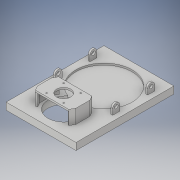
# Autodesk Inventor part: base
Saved by Autodesk Inventor 2019 (Build 230136000, 136)
## iProperties
Created: 2019-05-15
Part Number: base
Material: Generic
Document SubType Name: Modeling
Designer: Nathan
Density: 1 g/cm^3
Appearance: Default
Author: Nathan
Autodesk Inventor part; units mm, degrees
ref_plane "YZ Plane" through (0, 0, 0) normal (1, 0, 0) x (0, 1, 0)
ref_plane "XZ Plane" through (0, 0, 0) normal (0, 1, 0) x (-1, 0, 0)
ref_plane "XY Plane" through (0, 0, 0) normal (0, 0, 1) x (1, 0, 0)
sketch "Sketch1" plane through (0, 0, 0) normal (0, 1, 0) x (-1, 0, 0)
  line L0 (63.5, 88.9) -> (-63.5, 88.9)
  line L1 (-63.5, 88.9) -> (-63.5, -88.9)
  line L2 (-63.5, -88.9) -> (63.5, -88.9)
  line L3 (63.5, -88.9) -> (63.5, 88.9)
  line L4 (63.5, 88.9) -> (-63.5, -88.9) construction
  line L5 (-63.5, 88.9) -> (63.5, -88.9) construction
  point P0 (0, 0)
  dimension "d0" = 127
  dimension "d1" = 177.8
  constraints: 12 end point, 2 midpoint, 2 parallel, 1 horizontal, 1 perpendicular
  measures "d0" distance of L2.end L1.end
  measures "d1" distance of L1.end L0.end
extrude "Extrusion1" add sketch "Sketch1" along normal blind 12.7
sketch "Sketch2" plane through (0, 12.7, 0) normal (0, 1, 0) x (1, 0, 0)
  circle A0 centre (0, 25.4) radius 51.0159
  line L0 (-63.5, 88.9) -> (-63.5, -88.9) projected
  line L1 (63.5, 88.9) -> (-63.5, 88.9) projected
  point P0 (0, 0)
  dimension "d4" = 102.0318
  dimension "d5" = 63.5
  dimension "d6" = 63.5
  constraints: 1 centre point
  measures "d4" diameter of A0
  measures "d5" distance from line of L0 A0.centre
  measures "d6" distance from line of L1 A0.centre
sketch "Sketch3" plane through (0, 12.7, 0) normal (0, 1, 0) x (1, 0, 0)
  arc A0 (-24.2412, -32.7116) -> (24.2412, -32.7116) centre (0, -47.8409) ccw
  line L0 (-24.2412, -32.7116) -> (-17.8095, -22.4063)
  line L1 (0, 124.46) -> (0, -124.46) projected
  line L2 (24.2412, -32.7116) -> (17.8095, -22.4063)
  arc A1 (17.8095, -22.4063) -> (-17.8095, -22.4063) centre (0, -33.5215) ccw
  circle A2 centre (0, -47.8409) radius 22.225 construction
  circle A3 centre (0, 25.4) radius 51.0159 projected
  point P0 (0, 0)
  dimension "d13" = 57.15
  dimension "d14" = 70
  dimension "d58" = 44.45
  constraints: 4 end point, 4 point on circle, 3 centre point, 2 symmetric about line, 2 tangent, 1 coincident, 1 point on line, 1 vertical alignment, 1 other
  measures "d13" diameter of A0
  measures "d58" diameter of A2
extrude "Extrusion3" cut sketch "Sketch3" against normal through all contours L0 A3 L1 A0 | L1 A3 L2 A0 | A1 L1 A3 | L1 A1 A3 picked at (-3.4245, -21.2764) picked at (3.4245, -21.2764)
sketch "Sketch5" plane through (0, 12.7, 0) normal (0, 1, 0) x (1, 0, 0)
  line L0 (-34.925, -35.1409) -> (-30.2521, -26.8409)
  line L1 (-30.2521, -26.8409) -> (-27.4855, -28.3985)
  line L2 (-27.4855, -28.3985) -> (-31.75, -35.9732)
  line L3 (-31.75, -35.9732) -> (-31.75, -59.7086)
  line L4 (-31.75, -59.7086) -> (-27.4855, -67.2833)
  line L5 (-27.4855, -67.2833) -> (-30.2521, -68.8409)
  line L6 (-34.925, -35.1409) -> (-34.925, -60.5409)
  line L7 (-34.925, -60.5409) -> (-30.2521, -68.8409)
  arc A0 (-24.2412, -32.7116) -> (24.2412, -32.7116) centre (0, -47.8409) ccw projected
  arc A1 (-24.2412, -32.7116) -> (24.2412, -32.7116) centre (0, -47.8409) ccw construction
  line L8 (-28.575, -47.8409) -> (28.575, -47.8409) construction
  line L9 (0, 124.46) -> (0, -124.46) construction
  line L10 (34.925, -35.1409) -> (30.2521, -26.8409)
  line L11 (30.2521, -26.8409) -> (27.4855, -28.3985)
  line L12 (27.4855, -28.3985) -> (31.75, -35.9732)
  line L13 (31.75, -35.9732) -> (31.75, -59.7086)
  line L14 (31.75, -59.7086) -> (27.4855, -67.2833)
  line L15 (27.4855, -67.2833) -> (30.2521, -68.8409)
  line L16 (34.925, -35.1409) -> (34.925, -60.5409)
  line L17 (34.925, -60.5409) -> (30.2521, -68.8409)
  point P0 (0, 0)
  point P1 (-31.75, -47.8409)
  point P2 (31.75, -47.8409)
  dimension "d16" = 3.175
  dimension "d17" = 3.175
  dimension "d18" = 3.175
  dimension "d19" = 42
  dimension "d20" = 25.4
  dimension "d21" = 9.525
  dimension "d22" = 63.5
  constraints: 34 end point, 9 symmetric about line, 3 parallel, 2 midpoint, 2 point on circle, 1 coincident, 1 horizontal, 1 horizontal alignment, 1 perpendicular, 1 vertical, 2 other
  measures "d16" distance between parallel lines of L6 L3
  measures "d17" distance between parallel lines of L2 L0
  measures "d18" distance between parallel lines of L7 L4
  measures "d19" distance of L5.end L0.end
  measures "d20" distance of L0.start L6.end
  measures "d21" distance of L0.start L0.end
  measures "d22" distance between parallel lines of L13 L3
extrude "Extrusion4" add sketch "Sketch5" along normal blind 25.4
sketch "Sketch6" plane through (0, 38.1, 0) normal (0, 1, 0) x (1, 0, 0)
  line L0 (-30.2521, -68.8409) -> (-27.4855, -67.2833) projected
  line L1 (27.4855, -67.2833) -> (30.2521, -68.8409) projected
  line L2 (31.75, -59.7086) -> (27.4855, -67.2833) projected
  line L3 (31.75, -35.9732) -> (31.75, -59.7086) projected
  line L4 (27.4855, -28.3985) -> (31.75, -35.9732) projected
  line L5 (30.2521, -26.8409) -> (27.4855, -28.3985) projected
  line L6 (-27.4855, -28.3985) -> (-30.2521, -26.8409) projected
  line L7 (-31.75, -35.9732) -> (-27.4855, -28.3985) projected
  line L8 (-31.75, -59.7086) -> (-31.75, -35.9732) projected
  line L9 (-27.4855, -67.2833) -> (-31.75, -59.7086) projected
  line L10 (-30.2521, -68.8409) -> (30.2521, -68.8409)
  line L11 (30.2521, -26.8409) -> (-30.2521, -26.8409)
  point P0 (0, 0)
  constraints: 4 end point, 1 horizontal, 1 parallel
extrude "Extrusion5" add sketch "Sketch6" against normal blind 3.175
sketch "Sketch7" plane through (0, 38.1, 0) normal (0, 1, 0) x (1, 0, 0)
  arc A0 (-24.2412, -32.7116) -> (24.2412, -32.7116) centre (0, -47.8409) ccw projected
  line L0 (21, -68.8409) -> (-21, -68.8409) construction
  line L1 (-21, -68.8409) -> (-21, -26.8409) construction
  line L2 (-21, -26.8409) -> (21, -26.8409) construction
  line L3 (21, -26.8409) -> (21, -68.8409) construction
  line L4 (21, -68.8409) -> (-21, -26.8409) construction
  line L5 (-21, -68.8409) -> (21, -26.8409) construction
  line L6 (15.5, -63.3409) -> (-15.5, -63.3409) construction
  line L7 (-15.5, -63.3409) -> (-15.5, -32.3409) construction
  line L8 (-15.5, -32.3409) -> (15.5, -32.3409) construction
  line L9 (15.5, -32.3409) -> (15.5, -63.3409) construction
  line L10 (15.5, -63.3409) -> (-15.5, -32.3409) construction
  line L11 (-15.5, -63.3409) -> (15.5, -32.3409) construction
  circle A1 centre (0, -47.8409) radius 12.7
  point P0 (0, 0)
  dimension "d27" = 42
  dimension "d28" = 42
  dimension "d29" = 31
  dimension "d30" = 31
  dimension "d31" = 25.4
  constraints: 24 end point, 5 coincident, 4 midpoint, 4 parallel, 2 horizontal, 2 perpendicular, 1 centre point
  measures "d27" distance of L1.end L2.end
  measures "d28" distance of L0.end L1.end
  measures "d29" distance of L7.end L8.end
  measures "d30" distance of L6.end L7.end
  measures "d31" diameter of A1
extrude "Extrusion6" cut sketch "Sketch7" against normal through all
hole "Hole1" at (-15.5, 38.1, 63.3409) at (15.5, 38.1, 63.3409) at (15.5, 38.1, 32.3409) at (-15.5, 38.1, 32.3409) direction (0, -1, 0) diameter 2.5 depth 3.175 tip angle 118
sketch "Sketch8" plane through (0, 12.7, 0) normal (0, 1, 0) x (1, 0, 0)
  line L0 (-53.975, -12.7) -> (-50.8, -12.7)
  line L1 (-50.8, -12.7) -> (-50.8, 0)
  line L2 (-50.8, 0) -> (-53.975, 0)
  line L3 (-53.975, 0) -> (-53.975, -12.7)
  line L4 (-51.0159, 25.4) -> (51.0159, 25.4) construction
  line L5 (0, -25.6159) -> (0, 76.4159) construction
  point P0 (0, 0)
  point P1 (0, 25.4)
  point P2 (0, 25.4)
  dimension "d41" = 12.7
  dimension "d42" = 3.175
  dimension "d43" = 25.4
  dimension "d44" = 50.8
  constraints: 12 end point, 3 horizontal, 3 midpoint, 2 parallel, 2 perpendicular, 1 vertical, 3 other
  measures "d41" distance of L2.end L0.start
  measures "d42" distance of L0.start L0.end
  measures "d43" distance between parallel lines of L2 L4
  measures "d44" distance between parallel lines of L5 L1
extrude "Extrusion7" add sketch "Sketch8" along normal blind 10.287
sketch "Sketch9" plane through (-53.975, 12.7, 0) normal (-1, 0, 0) x (0, 0, 1)
  line L0 (12.7, 10.287) -> (0, 10.287) projected
  arc A0 (12.7, 10.287) -> (0, 10.287) centre (6.35, 10.287) ccw
  point P0 (0, -12.7)
  constraints: 2 end point, 2 point on circle, 1 centre point, 1 coincident, 1 midpoint
extrude "Extrusion8" add sketch "Sketch9" against normal blind 3.175
hole "Hole2" at (-53.975, 22.987, 6.35) direction (1, 0, 0) diameter 6.731 depth 3.175 tip angle 118
ref_plane "Work Plane1" through (-51.0159, 12.7, -25.4) normal (0, 0, 1) x (1, 0, 0)
ref_plane "Work Plane2" through (0, 12.7, 25.6159) normal (1, 0, 0) x (0, 0, -1)
mirror "Mirror1" about plane through (-51.0159, 12.7, -25.4) normal (0, 0, 1) of "Extrusion7", "Extrusion8", "Hole2"
mirror "Mirror2" about plane through (0, 12.7, 25.6159) normal (1, 0, 0) of "Extrusion7", "Extrusion8", "Hole2", "Mirror1"
extrude "Extrusion10" cut sketch "Sketch2" against normal blind 3.175
equation "\"d0\" = base_width"
equation "\"d1\" = base_length"
equation "\"d2\" = base_height"
equation "\"d6\" = d5"
equation "\"d14\" = base_cutout_contact_angle"
equation "\"d58\" = base_cutout_diameter"
equation "\"d11\" = turntable_bed_depth"
equation "\"d16\" = turntable_motor_support_thickness"
equation "\"d17\" = turntable_motor_support_thickness"
equation "\"d18\" = turntable_motor_support_thickness"
equation "\"d22\" = turntable_motor_support_width"
equation "\"d23\" = turntable_motor_support_height"
equation "\"d25\" = turntable_motor_support_thickness"
equation "\"d31\" = turntable_motor_boss"
equation "\"d32\" = turntable_motor_support_thickness"
equation "\"d39\" = turntable_motor_support_thickness"
equation "\"d54\" = turntable_motor_support_thickness"
equation "\"d63\" = turntable_bed_depth"
equation "\"base_length\" = 177.8"
equation "\"base_width\" = 127"
equation "\"base_height\" = 12.7"
equation "\"turntable_diameter\" = 101.6"
equation "\"turntable_height\" = 9.525"
equation "\"turntable_spur_width\" = 6.35"
equation "\"spine_diameter\" = 31.75"
equation "\"spine_height\" = 25.4"
equation "\"shoulder_length\" = 50.8"
equation "\"shoulder_width\" = 69.85"
equation "\"shoulder_wall_thickness\" = 4.7625"
equation "\"shoulder_gear_diameter\" = 63.5"
equation "\"shoulder_motor_gear_diameter\" = 25.4"
equation "\"shoulder_gear_shaft_diameter\" = 12.7"
equation "\"shoulder_motor_boss\" = 25.4"
equation "\"turntable_bed_depth\" = 3.175"
equation "\"base_cutout_diameter\" = 44.45"
equation "\"base_turntable_contact_angle\" = 60deg"
equation "\"base_cutout_contact_angle\" = 70deg"
equation "\"turntable_motor_support_thickness\" = 3.175"
equation "\"turntable_motor_support_height\" = 25.4"
equation "\"turntable_motor_boss\" = 25.4"
equation "\"turntable_motor_support_width\" = 63.5"
equation "\"turntable_retention_shaft_diameter\" = 6.35"
equation "\"turntable_retention_shaft_length\" = 152.4"
equation "\"shoulder_gear_thickness\" = 6.35"
equation "\"arm_distal_length\" = 177.8"
equation "\"arm_proximal_length\" = 228.6"
equation "\"arm_proximal_central_diameter\" = 25.4"
equation "\"arm_proximal_thickness\" = 6.35"
equation "\"arm_proximal_motor_boss\" = 25.4"
equation "\"turntable_ring_height\" = 9.525"
equation "\"turntable_ring_diameter\" = 19.05"
body "Solid1"
